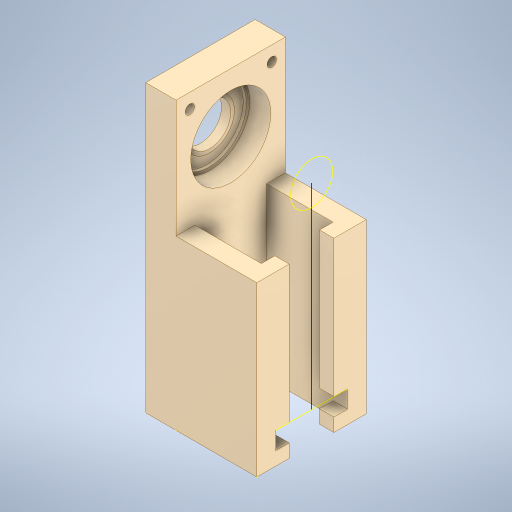
# Autodesk Inventor part: base
Saved by Autodesk Inventor 2023 (Build 270158000, 158)
## iProperties
Created: 2024-07-31
Part Number: base
Material: Generic
Document SubType Name: Modeling
Designer: sebas
Density: 1 g/cm^3
Appearance: Smooth - Off-White
Author: sebas
Autodesk Inventor part; units mm, degrees
ref_plane "YZ Plane" through (0, 0, 0) normal (1, 0, 0) x (0, 1, 0)
ref_plane "XZ Plane" through (0, 0, 0) normal (0, 1, 0) x (-1, 0, 0)
ref_plane "XY Plane" through (0, 0, 0) normal (0, 0, 1) x (1, 0, 0)
sketch "Sketch3" plane through (0, 0, 0) normal (0, 1, 0) x (-1, 0, 0)
  line L0 (0, 0) -> (0, -65)
  line L1 (0, -65) -> (25, -65)
  line L2 (25, -65) -> (25, 0)
  line L3 (25, 0) -> (0, 0)
  dimension "d8" = 65
  dimension "d9" = 25
  dimension "d10" = 65
  constraints: 8 end point, 2 perpendicular, 1 vertical
  measures "d8" distance of L0.start L0.end
  measures "d9" distance of L0.end L1.end
  measures "d10" distance of L1.end L2.end
extrude "Extrusion2" add sketch "Sketch3" along normal blind 170
sketch "Sketch4" plane through (0, 0, 0) normal (1, 0, 0) x (0, 0, -1)
  line L0 (65, 170) -> (0, 170) projected
  line L1 (0, 170) -> (32.5, 170)
  line L2 (65, 0) -> (65, 170) projected
  line L3 (32.5, 170) -> (32.5, 135)
  circle A0 centre (32.5, 135) radius 23.75
  point P0 (0, 0)
  dimension "d13" = 32.5
  dimension "d15" = 35
  dimension "d16" = 47.5
  constraints: 4 end point, 1 centre point, 1 coincident, 1 midpoint, 1 perpendicular
  measures "d13" distance of L0.end L1.end
  measures "d15" distance of L1.end L3.end
  measures "d16" diameter of A0
extrude "Extrusion3" cut sketch "Sketch4" against normal blind 12.5
sketch "Sketch6" plane through (0, 0, 0) normal (1, 0, 0) x (0, 0, -1)
  line L0 (65, 0) -> (0, 0) projected
  line L1 (0, 0) -> (32.5, 0)
  line L2 (32.5, 0) -> (11.2, 0)
  line L3 (11.2, 0) -> (53.8, 0)
  line L4 (53.8, 0) -> (53.8, 100)
  line L5 (53.8, 100) -> (65, 100)
  line L6 (65, 0) -> (65, 170) projected
  line L7 (65, 0) -> (53.8, 0)
  line L8 (11.2, 0) -> (0, 0)
  line L9 (0, 0) -> (0, 170) projected
  line L10 (0, 100) -> (11.2, 100)
  line L11 (11.2, 100) -> (11.2, 0)
  dimension "d23" = 21.3
  dimension "d24" = 42.6
  dimension "d25" = 100
  constraints: 18 end point, 6 point on line, 3 perpendicular, 1 collinear, 1 midpoint, 1 parallel
  measures "d23" distance of L1.end L2.end
  measures "d24" distance of L2.end L3.end
  measures "d25" distance of L3.end L4.end
extrude "Extrusion4" add sketch "Sketch6" along normal blind 39.5
sketch "Sketch7" plane through (39.5, 0, 0) normal (1, 0, 0) x (0, 0, -1)
  line L0 (65, 0) -> (0, 0) projected
  line L1 (53.8, 0) -> (53.8, 100) projected
  line L2 (65, 0) -> (53.8, 0)
  line L3 (53.8, 0) -> (45.8, 0)
  line L4 (45.8, 0) -> (45.8, 100)
  line L5 (53.8, 100) -> (65, 100) projected
  line L6 (45.8, 100) -> (65, 100)
  line L7 (65, 0) -> (65, 170) projected
  line L8 (65, 100) -> (65, 0)
  line L9 (11.2, 100) -> (11.2, 0) projected
  line L10 (11.2, 0) -> (19.2, 0)
  line L11 (19.2, 0) -> (19.2, 100)
  line L12 (0, 100) -> (11.2, 100) projected
  line L13 (19.2, 100) -> (0, 100)
  line L14 (0, 100) -> (0, 0)
  dimension "d28" = 8
  dimension "d29" = 8
  constraints: 18 end point, 5 perpendicular, 4 point on line, 1 collinear, 1 horizontal
  measures "d28" distance of L1.start L3.end
  measures "d29" distance of L9.end L10.end
extrude "Extrusion5" add sketch "Sketch7" along normal blind 8.5
sketch "Sketch8" plane through (48, 0, 0) normal (1, 0, 0) x (0, 0, -1)
  circle A0 centre (32.5, 135) radius 23.75 projected
  circle A1 centre (32.5, 135) radius 76.5
  line L0 (65, 0) -> (0, 0) projected
  line L1 (32.5, 0) -> (32.5, 58.5)
  line L2 (32.5, 58.5) -> (32.5, 57.9046)
  line L3 (32.5, 58.5) -> (32.5, 40.5)
  circle A2 centre (32.5, 49.5) radius 9
  line L4 (32.5, 49.5) -> (32.5, 28.5)
  line L5 (32.5, 28.5) -> (53.5, 28.5)
  line L6 (53.8, 0) -> (53.8, 100) projected
  line L7 (53.5, 28.5) -> (53.5, 70.5)
  line L8 (53.5, 70.5) -> (11.5, 70.5)
  line L9 (11.2, 100) -> (11.2, 0) projected
  line L10 (11.5, 70.5) -> (11.5, 28.5)
  line L11 (11.5, 28.5) -> (32.5, 28.5)
  line L12 (32.5, 28.5) -> (32.5, 16.4931)
  line L13 (32.5, 28.5) -> (32.5, 18.5)
  line L14 (32.5, 18.5) -> (55.5, 18.5)
  line L15 (55.5, 18.5) -> (55.5, 8)
  line L16 (55.5, 8) -> (9.5, 8)
  line L17 (9.5, 8) -> (9.5, 18.5)
  line L18 (9.5, 18.5) -> (32.5, 18.5)
  point P0 (11.2, 18.5)
  point P1 (11.2, 8)
  point P2 (53.8, 8)
  point P3 (53.8, 18.5)
  dimension "d32" = 153
  dimension "d33" = 18
  dimension "d34" = 21
  dimension "d38" = 42
  dimension "d39" = 42
  dimension "d42" = 42
  dimension "d43" = 10
  dimension "d44" = 23
  dimension "d45" = 10.5
  dimension "d46" = 46
  dimension "d47" = 10.5
  constraints: 32 end point, 6 point on line, 4 perpendicular, 2 midpoint, 2 parallel, 2 vertical alignment, 1 coincident, 1 horizontal, 1 vertical, 4 other
  measures "d33" distance of L1.end L3.end
  measures "d34" distance of L4.start L4.end
  measures "d38" distance of L5.end L7.end
  measures "d39" distance of L7.end L8.end
  measures "d42" distance of L8.end L10.end
  measures "d43" distance of L4.end L13.end
  measures "d44" distance of L13.end L14.end
  measures "d45" distance of L14.end L15.end
  measures "d46" distance of L15.end L16.end
  measures "d47" distance of L16.end L17.end
extrude "Extrusion6" cut sketch "Sketch8" against normal through all contours L18 L1 L16 L9 | L6 L16 L1 L14
sketch "Sketch9" plane through (-12.5, 135, -32.5) normal (1, 0, 0) x (0, 0, -1)
  circle A0 centre (0, 0) radius 12.5
  point P0 (-32.5, -135)
  dimension "d50" = 25
  constraints: 1 centre point
  measures "d50" diameter of A0
extrude "Extrusion7" cut sketch "Sketch9" against normal through all
sketch "Sketch10" plane through (-25, 0, -65) normal (-1, 0, 0) x (0, 0, 1)
  line L0 (65, 0) -> (45.8, 0) projected
  line L1 (65, 0) -> (0, 0)
  line L2 (0, 0) -> (0, 170)
  line L3 (0, 170) -> (65, 170)
  line L4 (65, 170) -> (65, 0)
  constraints: 8 end point, 2 parallel, 1 horizontal, 1 perpendicular
extrude "Extrusion8" cut sketch "Sketch10" against normal blind 7
sketch "Sketch11" plane through (48, 0, 0) normal (1, 0, 0) x (0, 0, -1)
  circle A0 centre (32.5, 135) radius 12.5 projected
  line L0 (32.5, 135) -> (32.5, 18.5)
  line L1 (11.2, 18.5) -> (53.8, 18.5) projected
  point P0 (0, 0)
  constraints: 2 end point, 1 midpoint
sketch "Sketch12" plane through (-12.5, 135, -32.5) normal (1, 0, 0) x (0, 0, -1)
  circle A0 centre (0, 0) radius 12.5 projected
  circle A1 centre (0, 0) radius 14.65
  circle A2 centre (0, 0) radius 21.85
  point P0 (-32.5, -135)
  dimension "d55" = 29.3
  dimension "d56" = 43.7
  constraints: 2 centre point, 2 coincident
  measures "d55" diameter of A1
  measures "d56" diameter of A2
extrude "Extrusion9" cut sketch "Sketch12" against normal blind 2 contours A2
sketch "Sketch13" plane through (0, 170, 0) normal (1, 0, 0) x (0, 0, -1)
  line L0 (65, -170) -> (65, 0) projected
  circle A0 centre (32.5, -35) radius 21.85 projected
  line L1 (0, 0) -> (0, -170) projected
  circle A1 centre (32.5, -35) radius 14.65 projected
  circle A2 centre (32.5, -35) radius 23.75
  line L2 (65, 0) -> (48.6607, -17.5962)
  line L3 (16.3393, -17.5962) -> (0, 0)
  circle A3 centre (56.8304, -8.7981) radius 2.75
  circle A4 centre (8.1696, -8.7981) radius 2.75
  dimension "d59" = 5.5
  dimension "d60" = 5.5
  constraints: 4 end point, 3 centre point, 2 midpoint, 2 point on circle, 1 coincident
  measures "d59" diameter of A3
  measures "d60" diameter of A4
extrude "Extrusion10" cut sketch "Sketch13" against normal through all contours A4 L3 | L3 A4 | A3 L2 | L2 A3
sketch "Sketch14" plane through (0, 0, -11.2) normal (1, 0, 0) x (0, 0, -1)
  line L0 (0, 0) -> (42.6, 0) projected
  point P0 (-11.2, 0)
sketch "Sketch15" plane through (0, 0, -11.2) normal (1, 0, 0) x (0, 0, -1)
  line L0 (0, 0) -> (0, 8) projected
  line L1 (0, 0) -> (0, -8)
  line L2 (0, -8) -> (42.6, -8)
  line L3 (34.6, 0) -> (42.6, 0) projected
  line L4 (42.6, -8) -> (42.6, 0)
  line L5 (42.6, 0) -> (0, 0)
  point P0 (-11.2, 0)
  dimension "d63" = 8
  constraints: 8 end point, 3 perpendicular, 1 vertical
  measures "d63" distance of L0.start L1.end
extrude "Extrusion11" add sketch "Sketch15" against normal blind 18
sketch "Sketch16" plane through (0, 8, -11.2) normal (1, 0, 0) x (0, 0, -1)
  line L0 (0, -8) -> (8, -8) projected
  line L1 (8, -8) -> (12, -8)
  line L2 (42.6, -16) -> (0, -16) projected
  line L3 (34.6, 0) -> (34.6, -8) projected
  line L4 (12, -8) -> (34.6, -8)
  line L5 (34.6, -8) -> (29.6, -8)
  circle A0 centre (29.6, -8) radius 2.75
  circle A1 centre (12, -8) radius 2.75
  point P0 (-11.2, -8)
  dimension "d66" = 4
  dimension "d67" = 5
  dimension "d68" = 5.5
  dimension "d69" = 5.5
  constraints: 6 end point, 2 centre point, 2 coincident, 1 collinear, 1 parallel, 1 point on line
  measures "d66" distance of L0.end L1.end
  measures "d67" distance of L3.end L5.end
  measures "d68" diameter of A0
  measures "d69" diameter of A1
extrude "Extrusion12" cut sketch "Sketch16" against normal through all
sketch "Sketch17" plane through (0, 170, 0) normal (1, 0, 0) x (0, 0, -1)
  point P0 (0, -170)
sketch "Sketch18" plane through (-18, 0, -65) normal (-1, 0, 0) x (0, 0, 1)
  point P0 (65, 0)
sketch "Sketch19" plane through (-18, 0, -65) normal (-1, 0, 0) x (0, 0, 1)
  point P0 (65, 0)
body "Solid2"
